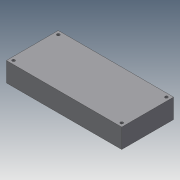
# Autodesk Inventor part: LCD
Saved by Autodesk Inventor 2014 SP1 (Build 180222100, 222)
## iProperties
Created: 2015-04-02
Part Number: LCD
Material: Generic
Document SubType Name: Modeling
Designer: tom
Density: 1 g/cm^3
Appearance: Default
Author: tom
Autodesk Inventor part; units mm, degrees
ref_plane "YZ Plane" through (0, 0, 0) normal (1, 0, 0) x (0, 1, 0)
ref_plane "XZ Plane" through (0, 0, 0) normal (0, 1, 0) x (-1, 0, 0)
ref_plane "XY Plane" through (0, 0, 0) normal (0, 0, 1) x (1, 0, 0)
sketch "Sketch1" plane through (0, 0, 0) normal (0, 1, 0) x (-1, 0, 0)
  line L0 (40, 18) -> (-40, 18)
  line L1 (-40, 18) -> (-40, -18)
  line L2 (-40, -18) -> (40, -18)
  line L3 (40, -18) -> (40, 18)
  circle A0 centre (37.5, -15.5) radius 1
  line L4 (37.5, -15.5) -> (-37.5, -15.5) construction
  line L5 (-37.5, -15.5) -> (-37.5, 15.5) construction
  line L6 (-37.5, 15.5) -> (37.5, 15.5) construction
  line L7 (37.5, 15.5) -> (37.5, -15.5) construction
  circle A1 centre (37.5, 15.5) radius 1
  circle A2 centre (-37.5, -15.5) radius 1
  circle A3 centre (-37.5, 15.5) radius 1
  point P0 (0, 0)
  dimension "d0" = 80
  dimension "d1" = 36
  dimension "d2" = 18
  dimension "d3" = 40
  dimension "d4" = 2
  dimension "d5" = 75
  dimension "d6" = 31
  dimension "d7" = 37.5
  dimension "d8" = 15.5
  dimension "d9" = 2
  dimension "d10" = 2
  dimension "d11" = 2
  constraints: 16 end point, 4 centre point, 4 coincident, 3 parallel, 3 perpendicular, 2 horizontal
  measures "d0" distance of L0.start L0.end
  measures "d1" distance of L0.end L1.end
  measures "d2" distance from line of point (0, 0) L0
  measures "d3" distance from line of point (0, 0) L1
  measures "d4" diameter of A0
  measures "d5" distance of L4.start L4.end
  measures "d6" distance of L6.end L4.start
  measures "d7" distance from line of point (0, 0) L5
  measures "d8" distance from line of point (0, 0) L6
  measures "d9" diameter of A1
  measures "d10" diameter of A2
  measures "d11" diameter of A3
extrude "Extrusion1" add sketch "Sketch1" along normal blind 13.5
equation "\"d2\" = 0.5 * d1"
equation "\"d3\" = 0.5 * d0"
equation "\"d7\" = 0.5 * d5"
equation "\"d8\" = 0.5 * d6"
body "Solid1"
